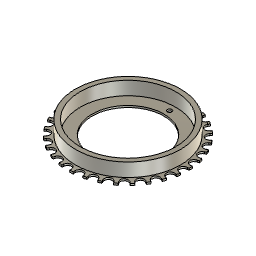
Big gear (Autodesk Fusion 360 design; units mm, degrees)
Autodesk Fusion 360 part; units mm, degrees
note: some values were not read from the file. Set by a fixed rule: which sketch regions a step uses.
sketch "Sketch1" plane through (0, 0, 0) normal (0, 1, 0) x (1, 0, 0)
sketch "Sketch2" plane through (0, 0, 0) normal (0, 0, 1) x (1, 0, 0)
  circle A0 centre (0, 0) radius 64.6805
  circle A1 centre (27.4355, 58.5735) radius 4.5
  circle A2 centre (15.4812, 62.8005) radius 4.5
  circle A3 centre (0, 0) radius 64.6805
  circle A4 centre (2.932, 64.614) radius 4.5
  circle A5 centre (0, 0) radius 64.6805
  circle A6 centre (-9.7299, 63.9445) radius 4.5
  circle A7 centre (0, 0) radius 64.6805
  circle A8 centre (-22.0179, 60.8176) radius 4.5
  circle A9 centre (0, 0) radius 64.6805
  circle A10 centre (-33.4597, 55.3535) radius 4.5
  circle A11 centre (0, 0) radius 64.6805
  circle A12 centre (-43.6158, 47.7623) radius 4.5
  circle A13 centre (0, 0) radius 64.6805
  circle A14 centre (-52.0956, 38.3355) radius 4.5
  circle A15 centre (0, 0) radius 64.6805
  circle A16 centre (-58.5735, 27.4355) radius 4.5
  circle A17 centre (0, 0) radius 64.6805
  circle A18 centre (-62.8005, 15.4812) radius 4.5
  circle A19 centre (0, 0) radius 64.6805
  circle A20 centre (-64.614, 2.932) radius 4.5
  circle A21 centre (0, 0) radius 64.6805
  circle A22 centre (-63.9445, -9.7299) radius 4.5
  circle A23 centre (-60.8176, -22.0179) radius 4.5
  circle A24 centre (0, 0) radius 64.6805
  circle A25 centre (-55.3535, -33.4597) radius 4.5
  circle A26 centre (0, 0) radius 64.6805
  circle A27 centre (-47.7623, -43.6158) radius 4.5
  circle A28 centre (0, 0) radius 64.6805
  circle A29 centre (-38.3355, -52.0956) radius 4.5
  circle A30 centre (-27.4355, -58.5735) radius 4.5
  circle A31 centre (0, 0) radius 64.6805
  circle A32 centre (-15.4812, -62.8005) radius 4.5
  circle A33 centre (0, 0) radius 64.6805
  circle A34 centre (-2.932, -64.614) radius 4.5
  circle A35 centre (0, 0) radius 64.6805
  circle A36 centre (9.7299, -63.9445) radius 4.5
  circle A37 centre (0, 0) radius 64.6805
  circle A38 centre (22.0179, -60.8176) radius 4.5
  circle A39 centre (0, 0) radius 64.6805
  circle A40 centre (33.4597, -55.3535) radius 4.5
  circle A41 centre (0, 0) radius 64.6805
  circle A42 centre (43.6158, -47.7623) radius 4.5
  circle A43 centre (0, 0) radius 64.6805
  circle A44 centre (52.0956, -38.3355) radius 4.5
  circle A45 centre (0, 0) radius 64.6805
  circle A46 centre (58.5735, -27.4355) radius 4.5
  circle A47 centre (0, 0) radius 64.6805
  circle A48 centre (62.8005, -15.4812) radius 4.5
  circle A49 centre (0, 0) radius 64.6805
  circle A50 centre (64.614, -2.932) radius 4.5
  circle A51 centre (0, 0) radius 64.6805
  circle A52 centre (63.9445, 9.7299) radius 4.5
  circle A53 centre (0, 0) radius 64.6805
  circle A54 centre (60.8176, 22.0179) radius 4.5
  circle A55 centre (0, 0) radius 64.6805
  circle A56 centre (55.3535, 33.4597) radius 4.5
  circle A57 centre (0, 0) radius 64.6805
  circle A58 centre (47.7623, 43.6158) radius 4.5
  circle A59 centre (0, 0) radius 64.6805
  circle A60 centre (38.3355, 52.0956) radius 4.5
  circle A61 centre (0, 0) radius 64.6805
  line L0 (31.4418, 56.5242) -> (34.7024, 54.583)
  line L1 (31.4418, 56.5242) -> (34.7024, 54.583)
  line L2 (31.4418, 56.5242) -> (32.4649, 58.2427)
  line L3 (32.4649, 58.2427) -> (35.6253, 56.3612)
  line L4 (35.6253, 56.3612) -> (34.5825, 54.6591)
  line L5 (19.8103, 61.5721) -> (20.4785, 63.4571)
  line L6 (20.4785, 63.4571) -> (23.9452, 62.2284)
  line L7 (23.9452, 62.2284) -> (23.2546, 60.3555)
  line L8 (7.4176, 64.2538) -> (7.7051, 66.233)
  line L9 (7.7051, 66.233) -> (11.3449, 65.7042)
  line L10 (11.3449, 65.7042) -> (11.033, 63.7326)
  line L11 (-5.2602, 64.4662) -> (-5.3643, 66.4635)
  line L12 (-5.3643, 66.4635) -> (-1.6913, 66.655)
  line L13 (-1.6913, 66.655) -> (-1.6126, 64.6604)
  line L14 (-17.7359, 62.2013) -> (-18.2277, 64.1399)
  line L15 (-18.2277, 64.1399) -> (-14.6626, 65.0443)
  line L16 (-14.6626, 65.0443) -> (-14.1963, 63.1034)
  line L17 (-29.53, 57.546) -> (-30.3905, 59.3515)
  line L18 (-30.3905, 59.3515) -> (-27.0703, 60.9339)
  line L19 (-27.0703, 60.9339) -> (-26.2343, 59.1213)
  line L20 (-40.1893, 50.6793) -> (-41.3855, 52.2821)
  line L21 (-41.3855, 52.2821) -> (-38.4378, 54.482)
  line L22 (-38.4378, 54.482) -> (-37.2642, 52.8672)
  line L23 (-49.3041, 41.865) -> (-50.79, 43.2036)
  line L24 (-50.79, 43.2036) -> (-48.3281, 45.9363)
  line L25 (-48.3281, 45.9363) -> (-46.8621, 44.5815)
  line L26 (-56.5242, 31.4418) -> (-58.2427, 32.4649)
  line L27 (-58.2427, 32.4649) -> (-56.3612, 35.6253)
  line L28 (-56.3612, 35.6253) -> (-54.6591, 34.5825)
  line L29 (-61.5721, 19.8103) -> (-63.4571, 20.4785)
  line L30 (-63.4571, 20.4785) -> (-62.2284, 23.9452)
  line L31 (-62.2284, 23.9452) -> (-60.3555, 23.2546)
  line L32 (-64.2538, 7.4176) -> (-66.233, 7.7051)
  line L33 (-66.233, 7.7051) -> (-65.7042, 11.3449)
  line L34 (-65.7042, 11.3449) -> (-63.7326, 11.033)
  line L35 (-64.4662, -5.2602) -> (-66.4635, -5.3643)
  line L36 (-66.4635, -5.3643) -> (-66.655, -1.6913)
  line L37 (-66.655, -1.6913) -> (-64.6604, -1.6126)
  line L38 (-62.2013, -17.7359) -> (-64.1399, -18.2277)
  line L39 (-64.1399, -18.2277) -> (-65.0443, -14.6626)
  line L40 (-65.0443, -14.6626) -> (-63.1034, -14.1963)
  line L41 (-57.546, -29.53) -> (-59.3515, -30.3905)
  line L42 (-59.3515, -30.3905) -> (-60.9339, -27.0703)
  line L43 (-60.9339, -27.0703) -> (-59.1213, -26.2343)
  line L44 (-50.6793, -40.1893) -> (-52.2821, -41.3855)
  line L45 (-52.2821, -41.3855) -> (-54.482, -38.4378)
  line L46 (-54.482, -38.4378) -> (-52.8672, -37.2642)
  line L47 (-41.865, -49.3041) -> (-43.2036, -50.79)
  line L48 (-43.2036, -50.79) -> (-45.9363, -48.3281)
  line L49 (-45.9363, -48.3281) -> (-44.5815, -46.8621)
  line L50 (-31.4418, -56.5242) -> (-32.4649, -58.2427)
  line L51 (-32.4649, -58.2427) -> (-35.6253, -56.3612)
  line L52 (-35.6253, -56.3612) -> (-34.5825, -54.6591)
  line L53 (-19.8103, -61.5721) -> (-20.4785, -63.4571)
  line L54 (-20.4785, -63.4571) -> (-23.9452, -62.2284)
  line L55 (-23.9452, -62.2284) -> (-23.2546, -60.3555)
  line L56 (-7.4176, -64.2538) -> (-7.7051, -66.233)
  line L57 (-7.7051, -66.233) -> (-11.3449, -65.7042)
  line L58 (-11.3449, -65.7042) -> (-11.033, -63.7326)
  line L59 (5.2602, -64.4662) -> (5.3643, -66.4635)
  line L60 (5.3643, -66.4635) -> (1.6913, -66.655)
  line L61 (1.6913, -66.655) -> (1.6126, -64.6604)
  line L62 (17.7359, -62.2013) -> (18.2277, -64.1399)
  line L63 (18.2277, -64.1399) -> (14.6626, -65.0443)
  line L64 (14.6626, -65.0443) -> (14.1963, -63.1034)
  line L65 (29.53, -57.546) -> (30.3905, -59.3515)
  line L66 (30.3905, -59.3515) -> (27.0703, -60.9339)
  line L67 (27.0703, -60.9339) -> (26.2343, -59.1213)
  line L68 (40.1893, -50.6793) -> (41.3855, -52.2821)
  line L69 (41.3855, -52.2821) -> (38.4378, -54.482)
  line L70 (38.4378, -54.482) -> (37.2642, -52.8672)
  line L71 (49.3041, -41.865) -> (50.79, -43.2036)
  line L72 (50.79, -43.2036) -> (48.3281, -45.9363)
  line L73 (48.3281, -45.9363) -> (46.8621, -44.5815)
  line L74 (56.5242, -31.4418) -> (58.2427, -32.4649)
  line L75 (58.2427, -32.4649) -> (56.3612, -35.6253)
  line L76 (56.3612, -35.6253) -> (54.6591, -34.5825)
  line L77 (61.5721, -19.8103) -> (63.4571, -20.4785)
  line L78 (63.4571, -20.4785) -> (62.2284, -23.9452)
  line L79 (62.2284, -23.9452) -> (60.3555, -23.2546)
  line L80 (64.2538, -7.4176) -> (66.233, -7.7051)
  line L81 (66.233, -7.7051) -> (65.7042, -11.3449)
  line L82 (65.7042, -11.3449) -> (63.7326, -11.033)
  line L83 (64.4662, 5.2602) -> (66.4635, 5.3643)
  line L84 (66.4635, 5.3643) -> (66.655, 1.6913)
  line L85 (66.655, 1.6913) -> (64.6604, 1.6126)
  line L86 (62.2013, 17.7359) -> (64.1399, 18.2277)
  line L87 (64.1399, 18.2277) -> (65.0443, 14.6626)
  line L88 (65.0443, 14.6626) -> (63.1034, 14.1963)
  line L89 (57.546, 29.53) -> (59.3515, 30.3905)
  line L90 (59.3515, 30.3905) -> (60.9339, 27.0703)
  line L91 (60.9339, 27.0703) -> (59.1213, 26.2343)
  line L92 (50.6793, 40.1893) -> (52.2821, 41.3855)
  line L93 (52.2821, 41.3855) -> (54.482, 38.4378)
  line L94 (54.482, 38.4378) -> (52.8672, 37.2642)
  line L95 (41.865, 49.3041) -> (43.2036, 50.79)
  line L96 (43.2036, 50.79) -> (45.9363, 48.3281)
  line L97 (45.9363, 48.3281) -> (44.5815, 46.8621)
  dimension "d1" = 129.361
  dimension "d2" = 9
  dimension "d4" = 360
  dimension "d6" = 2
  dimension "d8" = 360
  constraint coincident A0.centre A3.centre
  constraint coincident A0 A1.centre
  constraint coincident A33 L0.start
  constraint coincident A1 L0.start
  constraint coincident A31 L0.end
  constraint coincident A28 L0.end
  constraint perpendicular L1 L2
  constraint perpendicular L2 L3
  constraint coincident A59 L4.end
  constraint coincident A13 L4.end
  measures "d1" diameter of A0
  measures "d2" diameter of A1
  measures "d6" distance of L0.start L2.end
extrude "Extrude1" add sketch "Sketch2" along normal blind 2 contours A0 A1 A2 A3 A4 A5 A6 A7 A8 A9 A10 A11 A12 A13 A14 A15 A16 A17 A18 A19 A20 A21 A22 A23 A24 A25 A26 A27 A28 A29 A30 A31 A32 A33 A34 A35 A36 A37 A38 A39 A40 A41 A42 A43 A44 A45 A46 A47 A48 A49 A50 A51 A52 A53 A54 A55 A56 A57 A58 A59 A60 A61 L0 L1 | A0 A3 A5 A7 A9 A11 A13 A15 A17 A19 A21 A24 A26 A28 A31 A33 A35 A37 A39 A41 A43 A45 A47 A49 A51 A53 A55 A57 A59 A61 L83 L84 L85 | A0 A3 A5 A7 A9 A11 A13 A15 A17 A19 A21 A24 A26 A28 A31 A33 A35 A37 A39 A41 A43 A45 A47 A49 A51 A53 A55 A57 A59 A61 L80 L81 L82 | A0 A3 A5 A7 A9 A11 A13 A15 A17 A19 A21 A24 A26 A28 A31 A33 A35 A37 A39 A41 A43 A45 A47 A49 A51 A53 A55 A57 A59 A61 L86 L87 L88 | A0 A3 A5 A7 A9 A11 A13 A15 A17 A19 A21 A24 A26 A28 A31 A33 A35 A37 A39 A41 A43 A45 A47 A49 A51 A53 A55 A57 A59 A61 L77 L78 L79 | A0 A3 A5 A7 A9 A11 A13 A15 A17 A19 A21 A24 A26 A28 A31 A33 A35 A37 A39 A41 A43 A45 A47 A49 A51 A53 A55 A57 A59 A61 L89 L90 L91 | A0 A3 A5 A7 A9 A11 A13 A15 A17 A19 A21 A24 A26 A28 A31 A33 A35 A37 A39 A41 A43 A45 A47 A49 A51 A53 A55 A57 A59 A61 L74 L75 L76 | A0 A3 A5 A7 A9 A11 A13 A15 A17 A19 A21 A24 A26 A28 A31 A33 A35 A37 A39 A41 A43 A45 A47 A49 A51 A53 A55 A57 A59 A61 L92 L93 L94 | A0 A3 A5 A7 A9 A11 A13 A15 A17 A19 A21 A24 A26 A28 A31 A33 A35 A37 A39 A41 A43 A45 A47 A49 A51 A53 A55 A57 A59 A61 L71 L72 L73 | A0 A3 A5 A7 A9 A11 A13 A15 A17 A19 A21 A24 A26 A28 A31 A33 A35 A37 A39 A41 A43 A45 A47 A49 A51 A53 A55 A57 A59 A61 L95 L96 L97 | A0 A3 A5 A7 A9 A11 A13 A15 A17 A19 A21 A24 A26 A28 A31 A33 A35 A37 A39 A41 A43 A45 A47 A49 A51 A53 A55 A57 A59 A61 L68 L69 L70 | A0 A3 A5 A7 A9 A11 A13 A15 A17 A19 A21 A24 A26 A28 A31 A33 A35 A37 A39 A41 A43 A45 A47 A49 A51 A53 A55 A57 A59 A61 L2 L3 L4 | A0 A3 A5 A7 A9 A11 A13 A15 A17 A19 A21 A24 A26 A28 A31 A33 A35 A37 A39 A41 A43 A45 A47 A49 A51 A53 A55 A57 A59 A61 L5 L6 L7 | A0 A3 A5 A7 A9 A11 A13 A15 A17 A19 A21 A24 A26 A28 A31 A33 A35 A37 A39 A41 A43 A45 A47 A49 A51 A53 A55 A57 A59 A61 L65 L66 L67 | A0 A3 A5 A7 A9 A11 A13 A15 A17 A19 A21 A24 A26 A28 A31 A33 A35 A37 A39 A41 A43 A45 A47 A49 A51 A53 A55 A57 A59 A61 L8 L9 L10 | A0 A3 A5 A7 A9 A11 A13 A15 A17 A19 A21 A24 A26 A28 A31 A33 A35 A37 A39 A41 A43 A45 A47 A49 A51 A53 A55 A57 A59 A61 L62 L63 L64 | A0 A3 A5 A7 A9 A11 A13 A15 A17 A19 A21 A24 A26 A28 A31 A33 A35 A37 A39 A41 A43 A45 A47 A49 A51 A53 A55 A57 A59 A61 L11 L12 L13 | A0 A3 A5 A7 A9 A11 A13 A15 A17 A19 A21 A24 A26 A28 A31 A33 A35 A37 A39 A41 A43 A45 A47 A49 A51 A53 A55 A57 A59 A61 L59 L60 L61 | A0 A3 A5 A7 A9 A11 A13 A15 A17 A19 A21 A24 A26 A28 A31 A33 A35 A37 A39 A41 A43 A45 A47 A49 A51 A53 A55 A57 A59 A61 L14 L15 L16 | A0 A3 A5 A7 A9 A11 A13 A15 A17 A19 A21 A24 A26 A28 A31 A33 A35 A37 A39 A41 A43 A45 A47 A49 A51 A53 A55 A57 A59 A61 L56 L57 L58 | A0 A3 A5 A7 A9 A11 A13 A15 A17 A19 A21 A24 A26 A28 A31 A33 A35 A37 A39 A41 A43 A45 A47 A49 A51 A53 A55 A57 A59 A61 L17 L18 L19 | A0 A3 A5 A7 A9 A11 A13 A15 A17 A19 A21 A24 A26 A28 A31 A33 A35 A37 A39 A41 A43 A45 A47 A49 A51 A53 A55 A57 A59 A61 L53 L54 L55 | A0 A3 A5 A7 A9 A11 A13 A15 A17 A19 A21 A24 A26 A28 A31 A33 A35 A37 A39 A41 A43 A45 A47 A49 A51 A53 A55 A57 A59 A61 L20 L21 L22 | A0 A3 A5 A7 A9 A11 A13 A15 A17 A19 A21 A24 A26 A28 A31 A33 A35 A37 A39 A41 A43 A45 A47 A49 A51 A53 A55 A57 A59 A61 L50 L51 L52 | A0 A3 A5 A7 A9 A11 A13 A15 A17 A19 A21 A24 A26 A28 A31 A33 A35 A37 A39 A41 A43 A45 A47 A49 A51 A53 A55 A57 A59 A61 L23 L24 L25 | A0 A3 A5 A7 A9 A11 A13 A15 A17 A19 A21 A24 A26 A28 A31 A33 A35 A37 A39 A41 A43 A45 A47 A49 A51 A53 A55 A57 A59 A61 L47 L48 L49 | A0 A3 A5 A7 A9 A11 A13 A15 A17 A19 A21 A24 A26 A28 A31 A33 A35 A37 A39 A41 A43 A45 A47 A49 A51 A53 A55 A57 A59 A61 L26 L27 L28 | A0 A3 A5 A7 A9 A11 A13 A15 A17 A19 A21 A24 A26 A28 A31 A33 A35 A37 A39 A41 A43 A45 A47 A49 A51 A53 A55 A57 A59 A61 L44 L45 L46 | A0 A3 A5 A7 A9 A11 A13 A15 A17 A19 A21 A24 A26 A28 A31 A33 A35 A37 A39 A41 A43 A45 A47 A49 A51 A53 A55 A57 A59 A61 L29 L30 L31 | A0 A3 A5 A7 A9 A11 A13 A15 A17 A19 A21 A24 A26 A28 A31 A33 A35 A37 A39 A41 A43 A45 A47 A49 A51 A53 A55 A57 A59 A61 L41 L42 L43 | A0 A3 A5 A7 A9 A11 A13 A15 A17 A19 A21 A24 A26 A28 A31 A33 A35 A37 A39 A41 A43 A45 A47 A49 A51 A53 A55 A57 A59 A61 L32 L33 L34 | A0 A3 A5 A7 A9 A11 A13 A15 A17 A19 A21 A24 A26 A28 A31 A33 A35 A37 A39 A41 A43 A45 A47 A49 A51 A53 A55 A57 A59 A61 L38 L39 L40 | A0 A3 A5 A7 A9 A11 A13 A15 A17 A19 A21 A24 A26 A28 A31 A33 A35 A37 A39 A41 A43 A45 A47 A49 A51 A53 A55 A57 A59 A61 L35 L36 L37 makes body 1 at (-8.6099, -18.1233, 0)
sketch "Sketch9" plane through (0, 0, 2) normal (0, 0, 1) x (-1, 0, 0)
  arc A0 (-23.2965, -60.3394) -> (-23.2546, -60.3555) centre (0, 0) ccw
  line L0 (-23.2546, -60.3555) -> (-23.9452, -62.2284)
  line L1 (-23.9452, -62.2284) -> (-20.4785, -63.4571)
  line L2 (-20.4785, -63.4571) -> (-19.8103, -61.5721)
  arc A1 (-11.0772, -63.7249) -> (-19.8103, -61.5721) centre (-15.4812, -62.8005) ccw
  arc A2 (-11.0772, -63.7249) -> (-11.033, -63.7326) centre (0, 0) ccw
  line L3 (-11.033, -63.7326) -> (-11.3449, -65.7042)
  line L4 (-11.3449, -65.7042) -> (-7.7051, -66.233)
  line L5 (-7.7051, -66.233) -> (-7.4176, -64.2538)
  arc A3 (1.5677, -64.6615) -> (-7.4176, -64.2538) centre (-2.932, -64.614) ccw
  arc A4 (1.5677, -64.6615) -> (1.6126, -64.6604) centre (0, 0) ccw
  line L6 (1.6126, -64.6604) -> (1.6913, -66.655)
  line L7 (1.6913, -66.655) -> (5.3643, -66.4635)
  line L8 (5.3643, -66.4635) -> (5.2602, -64.4662)
  arc A5 (14.1524, -63.1132) -> (5.2602, -64.4662) centre (9.7299, -63.9445) ccw
  arc A6 (14.1524, -63.1132) -> (14.1963, -63.1034) centre (0, 0) ccw
  line L9 (14.1963, -63.1034) -> (14.6626, -65.0443)
  line L10 (14.6626, -65.0443) -> (18.2277, -64.1399)
  line L11 (18.2277, -64.1399) -> (17.7359, -62.2013)
  arc A7 (26.1933, -59.1395) -> (17.7359, -62.2013) centre (22.0179, -60.8176) ccw
  arc A8 (26.1933, -59.1395) -> (26.2343, -59.1213) centre (0, 0) ccw
  line L12 (26.2343, -59.1213) -> (27.0703, -60.9339)
  line L13 (27.0703, -60.9339) -> (30.3905, -59.3515)
  line L14 (30.3905, -59.3515) -> (29.53, -57.546)
  arc A9 (37.2275, -52.8931) -> (29.53, -57.546) centre (33.4597, -55.3535) ccw
  arc A10 (37.2275, -52.8931) -> (37.2642, -52.8672) centre (0, 0) ccw
  line L15 (37.2642, -52.8672) -> (38.4378, -54.482)
  line L16 (38.4378, -54.482) -> (41.3855, -52.2821)
  line L17 (41.3855, -52.2821) -> (40.1893, -50.6793)
  arc A11 (46.8311, -44.614) -> (40.1893, -50.6793) centre (43.6158, -47.7623) ccw
  arc A12 (46.8311, -44.614) -> (46.8621, -44.5815) centre (0, 0) ccw
  line L18 (46.8621, -44.5815) -> (48.3281, -45.9363)
  line L19 (48.3281, -45.9363) -> (50.79, -43.2036)
  line L20 (50.79, -43.2036) -> (49.3041, -41.865)
  arc A13 (54.6351, -34.6205) -> (49.3041, -41.865) centre (52.0956, -38.3355) ccw
  arc A14 (54.6351, -34.6205) -> (54.6591, -34.5825) centre (0, 0) ccw
  line L21 (54.6591, -34.5825) -> (56.3612, -35.6253)
  line L22 (56.3612, -35.6253) -> (58.2427, -32.4649)
  line L23 (58.2427, -32.4649) -> (56.5242, -31.4418)
  arc A15 (60.3394, -23.2965) -> (56.5242, -31.4418) centre (58.5735, -27.4355) ccw
  arc A16 (60.3394, -23.2965) -> (60.3555, -23.2546) centre (0, 0) ccw
  line L24 (60.3555, -23.2546) -> (62.2284, -23.9452)
  line L25 (62.2284, -23.9452) -> (63.4571, -20.4785)
  line L26 (63.4571, -20.4785) -> (61.5721, -19.8103)
  arc A17 (63.7249, -11.0772) -> (61.5721, -19.8103) centre (62.8005, -15.4812) ccw
  arc A18 (63.7249, -11.0772) -> (63.7326, -11.033) centre (0, 0) ccw
  line L27 (63.7326, -11.033) -> (65.7042, -11.3449)
  line L28 (65.7042, -11.3449) -> (66.233, -7.7051)
  line L29 (66.233, -7.7051) -> (64.2538, -7.4176)
  arc A19 (64.6615, 1.5677) -> (64.2538, -7.4176) centre (64.614, -2.932) ccw
  arc A20 (64.6615, 1.5677) -> (64.6604, 1.6126) centre (0, 0) ccw
  line L30 (64.6604, 1.6126) -> (66.655, 1.6913)
  line L31 (66.655, 1.6913) -> (66.4635, 5.3643)
  line L32 (66.4635, 5.3643) -> (64.4662, 5.2602)
  arc A21 (63.1132, 14.1524) -> (64.4662, 5.2602) centre (63.9445, 9.7299) ccw
  arc A22 (63.1132, 14.1524) -> (63.1034, 14.1963) centre (0, 0) ccw
  line L33 (63.1034, 14.1963) -> (65.0443, 14.6626)
  line L34 (65.0443, 14.6626) -> (64.1399, 18.2277)
  line L35 (64.1399, 18.2277) -> (62.2013, 17.7359)
  arc A23 (59.1395, 26.1933) -> (62.2013, 17.7359) centre (60.8176, 22.0179) ccw
  arc A24 (59.1395, 26.1933) -> (59.1213, 26.2343) centre (0, 0) ccw
  line L36 (59.1213, 26.2343) -> (60.9339, 27.0703)
  line L37 (60.9339, 27.0703) -> (59.3515, 30.3905)
  line L38 (59.3515, 30.3905) -> (57.546, 29.53)
  arc A25 (52.8931, 37.2275) -> (57.546, 29.53) centre (55.3535, 33.4597) ccw
  arc A26 (52.8931, 37.2275) -> (52.8672, 37.2642) centre (0, 0) ccw
  line L39 (52.8672, 37.2642) -> (54.482, 38.4378)
  line L40 (54.482, 38.4378) -> (52.2821, 41.3855)
  line L41 (52.2821, 41.3855) -> (50.6793, 40.1893)
  arc A27 (44.614, 46.8311) -> (50.6793, 40.1893) centre (47.7623, 43.6158) ccw
  arc A28 (44.614, 46.8311) -> (44.5815, 46.8621) centre (0, 0) ccw
  line L42 (44.5815, 46.8621) -> (45.9363, 48.3281)
  line L43 (45.9363, 48.3281) -> (43.2036, 50.79)
  line L44 (43.2036, 50.79) -> (41.865, 49.3041)
  arc A29 (34.6205, 54.6351) -> (41.865, 49.3041) centre (38.3355, 52.0956) ccw
  arc A30 (34.6205, 54.6351) -> (34.5825, 54.6591) centre (0, 0) ccw
  line L45 (34.5825, 54.6591) -> (35.6253, 56.3612)
  line L46 (35.6253, 56.3612) -> (32.4649, 58.2427)
  line L47 (32.4649, 58.2427) -> (31.4418, 56.5242)
  arc A31 (23.2965, 60.3394) -> (31.4418, 56.5242) centre (27.4355, 58.5735) ccw
  arc A32 (23.2965, 60.3394) -> (23.2546, 60.3555) centre (0, 0) ccw
  line L48 (23.2546, 60.3555) -> (23.9452, 62.2284)
  line L49 (23.9452, 62.2284) -> (20.4785, 63.4571)
  line L50 (20.4785, 63.4571) -> (19.8103, 61.5721)
  arc A33 (11.0772, 63.7249) -> (19.8103, 61.5721) centre (15.4812, 62.8005) ccw
  arc A34 (11.0772, 63.7249) -> (11.033, 63.7326) centre (0, 0) ccw
  line L51 (11.033, 63.7326) -> (11.3449, 65.7042)
  line L52 (11.3449, 65.7042) -> (7.7051, 66.233)
  line L53 (7.7051, 66.233) -> (7.4176, 64.2538)
  arc A35 (-1.5677, 64.6615) -> (7.4176, 64.2538) centre (2.932, 64.614) ccw
  arc A36 (-1.5677, 64.6615) -> (-1.6126, 64.6604) centre (0, 0) ccw
  line L54 (-1.6126, 64.6604) -> (-1.6913, 66.655)
  line L55 (-1.6913, 66.655) -> (-5.3643, 66.4635)
  line L56 (-5.3643, 66.4635) -> (-5.2602, 64.4662)
  arc A37 (-14.1524, 63.1132) -> (-5.2602, 64.4662) centre (-9.7299, 63.9445) ccw
  arc A38 (-14.1524, 63.1132) -> (-14.1963, 63.1034) centre (0, 0) ccw
  line L57 (-14.1963, 63.1034) -> (-14.6626, 65.0443)
  line L58 (-14.6626, 65.0443) -> (-18.2277, 64.1399)
  line L59 (-18.2277, 64.1399) -> (-17.7359, 62.2013)
  arc A39 (-26.1933, 59.1395) -> (-17.7359, 62.2013) centre (-22.0179, 60.8176) ccw
  arc A40 (-26.1933, 59.1395) -> (-26.2343, 59.1213) centre (0, 0) ccw
  line L60 (-26.2343, 59.1213) -> (-27.0703, 60.9339)
  line L61 (-27.0703, 60.9339) -> (-30.3905, 59.3515)
  line L62 (-30.3905, 59.3515) -> (-29.53, 57.546)
  arc A41 (-37.2275, 52.8931) -> (-29.53, 57.546) centre (-33.4597, 55.3535) ccw
  arc A42 (-37.2275, 52.8931) -> (-37.2642, 52.8672) centre (0, 0) ccw
  line L63 (-37.2642, 52.8672) -> (-38.4378, 54.482)
  line L64 (-38.4378, 54.482) -> (-41.3855, 52.2821)
  line L65 (-41.3855, 52.2821) -> (-40.1893, 50.6793)
  arc A43 (-46.8311, 44.614) -> (-40.1893, 50.6793) centre (-43.6158, 47.7623) ccw
  arc A44 (-46.8311, 44.614) -> (-46.8621, 44.5815) centre (0, 0) ccw
  line L66 (-46.8621, 44.5815) -> (-48.3281, 45.9363)
  line L67 (-48.3281, 45.9363) -> (-50.79, 43.2036)
  line L68 (-50.79, 43.2036) -> (-49.3041, 41.865)
  arc A45 (-54.6351, 34.6205) -> (-49.3041, 41.865) centre (-52.0956, 38.3355) ccw
  arc A46 (-54.6351, 34.6205) -> (-54.6591, 34.5825) centre (0, 0) ccw
  line L69 (-54.6591, 34.5825) -> (-56.3612, 35.6253)
  line L70 (-56.3612, 35.6253) -> (-58.2427, 32.4649)
  line L71 (-58.2427, 32.4649) -> (-56.5242, 31.4418)
  arc A47 (-60.3394, 23.2965) -> (-56.5242, 31.4418) centre (-58.5735, 27.4355) ccw
  arc A48 (-60.3394, 23.2965) -> (-60.3555, 23.2546) centre (0, 0) ccw
  line L72 (-60.3555, 23.2546) -> (-62.2284, 23.9452)
  line L73 (-62.2284, 23.9452) -> (-63.4571, 20.4785)
  line L74 (-63.4571, 20.4785) -> (-61.5721, 19.8103)
  arc A49 (-63.7249, 11.0772) -> (-61.5721, 19.8103) centre (-62.8005, 15.4812) ccw
  arc A50 (-63.7249, 11.0772) -> (-63.7326, 11.033) centre (0, 0) ccw
  line L75 (-63.7326, 11.033) -> (-65.7042, 11.3449)
  line L76 (-65.7042, 11.3449) -> (-66.233, 7.7051)
  line L77 (-66.233, 7.7051) -> (-64.2538, 7.4176)
  arc A51 (-64.6615, -1.5677) -> (-64.2538, 7.4176) centre (-64.614, 2.932) ccw
  arc A52 (-64.6615, -1.5677) -> (-64.6604, -1.6126) centre (0, 0) ccw
  line L78 (-64.6604, -1.6126) -> (-66.655, -1.6913)
  line L79 (-66.655, -1.6913) -> (-66.4635, -5.3643)
  line L80 (-66.4635, -5.3643) -> (-64.4662, -5.2602)
  arc A53 (-63.1132, -14.1524) -> (-64.4662, -5.2602) centre (-63.9445, -9.7299) ccw
  arc A54 (-63.1132, -14.1524) -> (-63.1034, -14.1963) centre (0, 0) ccw
  line L81 (-63.1034, -14.1963) -> (-65.0443, -14.6626)
  line L82 (-65.0443, -14.6626) -> (-64.1399, -18.2277)
  line L83 (-64.1399, -18.2277) -> (-62.2013, -17.7359)
  arc A55 (-59.1395, -26.1933) -> (-62.2013, -17.7359) centre (-60.8176, -22.0179) ccw
  arc A56 (-59.1395, -26.1933) -> (-59.1213, -26.2343) centre (0, 0) ccw
  line L84 (-59.1213, -26.2343) -> (-60.9339, -27.0703)
  line L85 (-60.9339, -27.0703) -> (-59.3515, -30.3905)
  line L86 (-59.3515, -30.3905) -> (-57.546, -29.53)
  arc A57 (-52.8931, -37.2275) -> (-57.546, -29.53) centre (-55.3535, -33.4597) ccw
  arc A58 (-52.8931, -37.2275) -> (-52.8672, -37.2642) centre (0, 0) ccw
  line L87 (-52.8672, -37.2642) -> (-54.482, -38.4378)
  line L88 (-54.482, -38.4378) -> (-52.2821, -41.3855)
  line L89 (-52.2821, -41.3855) -> (-50.6793, -40.1893)
  arc A59 (-44.614, -46.8311) -> (-50.6793, -40.1893) centre (-47.7623, -43.6158) ccw
  arc A60 (-44.614, -46.8311) -> (-44.5815, -46.8621) centre (0, 0) ccw
  line L90 (-44.5815, -46.8621) -> (-45.9363, -48.3281)
  line L91 (-45.9363, -48.3281) -> (-43.2036, -50.79)
  line L92 (-43.2036, -50.79) -> (-41.865, -49.3041)
  arc A61 (-34.6189, -54.6328) -> (-41.865, -49.3041) centre (-38.3355, -52.0956) ccw
  line L93 (-34.6189, -54.6328) -> (-31.4418, -56.5242)
  arc A62 (-23.2965, -60.3394) -> (-31.4418, -56.5242) centre (-27.4355, -58.5735) ccw
  circle A63 centre (0, 0) radius 40
  circle A64 centre (0, -46.5) radius 2.5
  circle A65 centre (0.1887, 46.5) radius 2.5
  dimension "d27" = 80
  dimension "d28" = 5
  dimension "d29" = 5
  dimension "d30" = 46.5
  dimension "d31" = 46.5
  constraint coincident A0.centre A2.centre
  measures "d27" diameter of A63
  measures "d28" diameter of A64
  measures "d29" diameter of A65
  measures "d30" distance of A0.centre A64.centre
  measures "d31" vertical distance of A0.centre A65.centre
extrude "Extrude7" cut sketch "Sketch9" against normal blind 3 contours A63 | A64 | A65 bodies 1
sketch "Sketch10" plane through (0, 0, 2) normal (0, 0, 1) x (-1, 0, 0)
  circle A0 centre (0, -46.5) radius 2.5
  circle A1 centre (0, 0) radius 40
  circle A2 centre (0.1887, 46.5) radius 2.5
  arc A3 (-23.2965, -60.3394) -> (-23.2546, -60.3555) centre (0, 0) ccw
  line L0 (-23.2546, -60.3555) -> (-23.9452, -62.2284)
  line L1 (-23.9452, -62.2284) -> (-20.4785, -63.4571)
  line L2 (-20.4785, -63.4571) -> (-19.8103, -61.5721)
  arc A4 (-11.0772, -63.7249) -> (-19.8103, -61.5721) centre (-15.4812, -62.8005) ccw
  arc A5 (-11.0772, -63.7249) -> (-11.033, -63.7326) centre (0, 0) ccw
  line L3 (-11.033, -63.7326) -> (-11.3449, -65.7042)
  line L4 (-11.3449, -65.7042) -> (-7.7051, -66.233)
  line L5 (-7.7051, -66.233) -> (-7.4176, -64.2538)
  arc A6 (1.5677, -64.6615) -> (-7.4176, -64.2538) centre (-2.932, -64.614) ccw
  arc A7 (1.5677, -64.6615) -> (1.6126, -64.6604) centre (0, 0) ccw
  line L6 (1.6126, -64.6604) -> (1.6913, -66.655)
  line L7 (1.6913, -66.655) -> (5.3643, -66.4635)
  line L8 (5.3643, -66.4635) -> (5.2602, -64.4662)
  arc A8 (14.1524, -63.1132) -> (5.2602, -64.4662) centre (9.7299, -63.9445) ccw
  arc A9 (14.1524, -63.1132) -> (14.1963, -63.1034) centre (0, 0) ccw
  line L9 (14.1963, -63.1034) -> (14.6626, -65.0443)
  line L10 (14.6626, -65.0443) -> (18.2277, -64.1399)
  line L11 (18.2277, -64.1399) -> (17.7359, -62.2013)
  arc A10 (26.1933, -59.1395) -> (17.7359, -62.2013) centre (22.0179, -60.8176) ccw
  arc A11 (26.1933, -59.1395) -> (26.2343, -59.1213) centre (0, 0) ccw
  line L12 (26.2343, -59.1213) -> (27.0703, -60.9339)
  line L13 (27.0703, -60.9339) -> (30.3905, -59.3515)
  line L14 (30.3905, -59.3515) -> (29.53, -57.546)
  arc A12 (37.2275, -52.8931) -> (29.53, -57.546) centre (33.4597, -55.3535) ccw
  arc A13 (37.2275, -52.8931) -> (37.2642, -52.8672) centre (0, 0) ccw
  line L15 (37.2642, -52.8672) -> (38.4378, -54.482)
  line L16 (38.4378, -54.482) -> (41.3855, -52.2821)
  line L17 (41.3855, -52.2821) -> (40.1893, -50.6793)
  arc A14 (46.8311, -44.614) -> (40.1893, -50.6793) centre (43.6158, -47.7623) ccw
  arc A15 (46.8311, -44.614) -> (46.8621, -44.5815) centre (0, 0) ccw
  line L18 (46.8621, -44.5815) -> (48.3281, -45.9363)
  line L19 (48.3281, -45.9363) -> (50.79, -43.2036)
  line L20 (50.79, -43.2036) -> (49.3041, -41.865)
  arc A16 (54.6351, -34.6205) -> (49.3041, -41.865) centre (52.0956, -38.3355) ccw
  arc A17 (54.6351, -34.6205) -> (54.6591, -34.5825) centre (0, 0) ccw
  line L21 (54.6591, -34.5825) -> (56.3612, -35.6253)
  line L22 (56.3612, -35.6253) -> (58.2427, -32.4649)
  line L23 (58.2427, -32.4649) -> (56.5242, -31.4418)
  arc A18 (60.3394, -23.2965) -> (56.5242, -31.4418) centre (58.5735, -27.4355) ccw
  arc A19 (60.3394, -23.2965) -> (60.3555, -23.2546) centre (0, 0) ccw
  line L24 (60.3555, -23.2546) -> (62.2284, -23.9452)
  line L25 (62.2284, -23.9452) -> (63.4571, -20.4785)
  line L26 (63.4571, -20.4785) -> (61.5721, -19.8103)
  arc A20 (63.7249, -11.0772) -> (61.5721, -19.8103) centre (62.8005, -15.4812) ccw
  arc A21 (63.7249, -11.0772) -> (63.7326, -11.033) centre (0, 0) ccw
  line L27 (63.7326, -11.033) -> (65.7042, -11.3449)
  line L28 (65.7042, -11.3449) -> (66.233, -7.7051)
  line L29 (66.233, -7.7051) -> (64.2538, -7.4176)
  arc A22 (64.6615, 1.5677) -> (64.2538, -7.4176) centre (64.614, -2.932) ccw
  arc A23 (64.6615, 1.5677) -> (64.6604, 1.6126) centre (0, 0) ccw
  line L30 (64.6604, 1.6126) -> (66.655, 1.6913)
  line L31 (66.655, 1.6913) -> (66.4635, 5.3643)
  line L32 (66.4635, 5.3643) -> (64.4662, 5.2602)
  arc A24 (63.1132, 14.1524) -> (64.4662, 5.2602) centre (63.9445, 9.7299) ccw
  arc A25 (63.1132, 14.1524) -> (63.1034, 14.1963) centre (0, 0) ccw
  line L33 (63.1034, 14.1963) -> (65.0443, 14.6626)
  line L34 (65.0443, 14.6626) -> (64.1399, 18.2277)
  line L35 (64.1399, 18.2277) -> (62.2013, 17.7359)
  arc A26 (59.1395, 26.1933) -> (62.2013, 17.7359) centre (60.8176, 22.0179) ccw
  arc A27 (59.1395, 26.1933) -> (59.1213, 26.2343) centre (0, 0) ccw
  line L36 (59.1213, 26.2343) -> (60.9339, 27.0703)
  line L37 (60.9339, 27.0703) -> (59.3515, 30.3905)
  line L38 (59.3515, 30.3905) -> (57.546, 29.53)
  arc A28 (52.8931, 37.2275) -> (57.546, 29.53) centre (55.3535, 33.4597) ccw
  arc A29 (52.8931, 37.2275) -> (52.8672, 37.2642) centre (0, 0) ccw
  line L39 (52.8672, 37.2642) -> (54.482, 38.4378)
  line L40 (54.482, 38.4378) -> (52.2821, 41.3855)
  line L41 (52.2821, 41.3855) -> (50.6793, 40.1893)
  arc A30 (44.614, 46.8311) -> (50.6793, 40.1893) centre (47.7623, 43.6158) ccw
  arc A31 (44.614, 46.8311) -> (44.5815, 46.8621) centre (0, 0) ccw
  line L42 (44.5815, 46.8621) -> (45.9363, 48.3281)
  line L43 (45.9363, 48.3281) -> (43.2036, 50.79)
  line L44 (43.2036, 50.79) -> (41.865, 49.3041)
  arc A32 (34.6205, 54.6351) -> (41.865, 49.3041) centre (38.3355, 52.0956) ccw
  arc A33 (34.6205, 54.6351) -> (34.5825, 54.6591) centre (0, 0) ccw
  line L45 (34.5825, 54.6591) -> (35.6253, 56.3612)
  line L46 (35.6253, 56.3612) -> (32.4649, 58.2427)
  line L47 (32.4649, 58.2427) -> (31.4418, 56.5242)
  arc A34 (23.2965, 60.3394) -> (31.4418, 56.5242) centre (27.4355, 58.5735) ccw
  arc A35 (23.2965, 60.3394) -> (23.2546, 60.3555) centre (0, 0) ccw
  line L48 (23.2546, 60.3555) -> (23.9452, 62.2284)
  line L49 (23.9452, 62.2284) -> (20.4785, 63.4571)
  line L50 (20.4785, 63.4571) -> (19.8103, 61.5721)
  arc A36 (11.0772, 63.7249) -> (19.8103, 61.5721) centre (15.4812, 62.8005) ccw
  arc A37 (11.0772, 63.7249) -> (11.033, 63.7326) centre (0, 0) ccw
  line L51 (11.033, 63.7326) -> (11.3449, 65.7042)
  line L52 (11.3449, 65.7042) -> (7.7051, 66.233)
  line L53 (7.7051, 66.233) -> (7.4176, 64.2538)
  arc A38 (-1.5677, 64.6615) -> (7.4176, 64.2538) centre (2.932, 64.614) ccw
  arc A39 (-1.5677, 64.6615) -> (-1.6126, 64.6604) centre (0, 0) ccw
  line L54 (-1.6126, 64.6604) -> (-1.6913, 66.655)
  line L55 (-1.6913, 66.655) -> (-5.3643, 66.4635)
  line L56 (-5.3643, 66.4635) -> (-5.2602, 64.4662)
  arc A40 (-14.1524, 63.1132) -> (-5.2602, 64.4662) centre (-9.7299, 63.9445) ccw
  arc A41 (-14.1524, 63.1132) -> (-14.1963, 63.1034) centre (0, 0) ccw
  line L57 (-14.1963, 63.1034) -> (-14.6626, 65.0443)
  line L58 (-14.6626, 65.0443) -> (-18.2277, 64.1399)
  line L59 (-18.2277, 64.1399) -> (-17.7359, 62.2013)
  arc A42 (-26.1933, 59.1395) -> (-17.7359, 62.2013) centre (-22.0179, 60.8176) ccw
  arc A43 (-26.1933, 59.1395) -> (-26.2343, 59.1213) centre (0, 0) ccw
  line L60 (-26.2343, 59.1213) -> (-27.0703, 60.9339)
  line L61 (-27.0703, 60.9339) -> (-30.3905, 59.3515)
  line L62 (-30.3905, 59.3515) -> (-29.53, 57.546)
  arc A44 (-37.2275, 52.8931) -> (-29.53, 57.546) centre (-33.4597, 55.3535) ccw
  arc A45 (-37.2275, 52.8931) -> (-37.2642, 52.8672) centre (0, 0) ccw
  line L63 (-37.2642, 52.8672) -> (-38.4378, 54.482)
  line L64 (-38.4378, 54.482) -> (-41.3855, 52.2821)
  line L65 (-41.3855, 52.2821) -> (-40.1893, 50.6793)
  arc A46 (-46.8311, 44.614) -> (-40.1893, 50.6793) centre (-43.6158, 47.7623) ccw
  arc A47 (-46.8311, 44.614) -> (-46.8621, 44.5815) centre (0, 0) ccw
  line L66 (-46.8621, 44.5815) -> (-48.3281, 45.9363)
  line L67 (-48.3281, 45.9363) -> (-50.79, 43.2036)
  line L68 (-50.79, 43.2036) -> (-49.3041, 41.865)
  arc A48 (-54.6351, 34.6205) -> (-49.3041, 41.865) centre (-52.0956, 38.3355) ccw
  arc A49 (-54.6351, 34.6205) -> (-54.6591, 34.5825) centre (0, 0) ccw
  line L69 (-54.6591, 34.5825) -> (-56.3612, 35.6253)
  line L70 (-56.3612, 35.6253) -> (-58.2427, 32.4649)
  line L71 (-58.2427, 32.4649) -> (-56.5242, 31.4418)
  arc A50 (-60.3394, 23.2965) -> (-56.5242, 31.4418) centre (-58.5735, 27.4355) ccw
  arc A51 (-60.3394, 23.2965) -> (-60.3555, 23.2546) centre (0, 0) ccw
  line L72 (-60.3555, 23.2546) -> (-62.2284, 23.9452)
  line L73 (-62.2284, 23.9452) -> (-63.4571, 20.4785)
  line L74 (-63.4571, 20.4785) -> (-61.5721, 19.8103)
  arc A52 (-63.7249, 11.0772) -> (-61.5721, 19.8103) centre (-62.8005, 15.4812) ccw
  arc A53 (-63.7249, 11.0772) -> (-63.7326, 11.033) centre (0, 0) ccw
  line L75 (-63.7326, 11.033) -> (-65.7042, 11.3449)
  line L76 (-65.7042, 11.3449) -> (-66.233, 7.7051)
  line L77 (-66.233, 7.7051) -> (-64.2538, 7.4176)
  arc A54 (-64.6615, -1.5677) -> (-64.2538, 7.4176) centre (-64.614, 2.932) ccw
  arc A55 (-64.6615, -1.5677) -> (-64.6604, -1.6126) centre (0, 0) ccw
  line L78 (-64.6604, -1.6126) -> (-66.655, -1.6913)
  line L79 (-66.655, -1.6913) -> (-66.4635, -5.3643)
  line L80 (-66.4635, -5.3643) -> (-64.4662, -5.2602)
  arc A56 (-63.1132, -14.1524) -> (-64.4662, -5.2602) centre (-63.9445, -9.7299) ccw
  arc A57 (-63.1132, -14.1524) -> (-63.1034, -14.1963) centre (0, 0) ccw
  line L81 (-63.1034, -14.1963) -> (-65.0443, -14.6626)
  line L82 (-65.0443, -14.6626) -> (-64.1399, -18.2277)
  line L83 (-64.1399, -18.2277) -> (-62.2013, -17.7359)
  arc A58 (-59.1395, -26.1933) -> (-62.2013, -17.7359) centre (-60.8176, -22.0179) ccw
  arc A59 (-59.1395, -26.1933) -> (-59.1213, -26.2343) centre (0, 0) ccw
  line L84 (-59.1213, -26.2343) -> (-60.9339, -27.0703)
  line L85 (-60.9339, -27.0703) -> (-59.3515, -30.3905)
  line L86 (-59.3515, -30.3905) -> (-57.546, -29.53)
  arc A60 (-52.8931, -37.2275) -> (-57.546, -29.53) centre (-55.3535, -33.4597) ccw
  arc A61 (-52.8931, -37.2275) -> (-52.8672, -37.2642) centre (0, 0) ccw
  line L87 (-52.8672, -37.2642) -> (-54.482, -38.4378)
  line L88 (-54.482, -38.4378) -> (-52.2821, -41.3855)
  line L89 (-52.2821, -41.3855) -> (-50.6793, -40.1893)
  arc A62 (-44.614, -46.8311) -> (-50.6793, -40.1893) centre (-47.7623, -43.6158) ccw
  arc A63 (-44.614, -46.8311) -> (-44.5815, -46.8621) centre (0, 0) ccw
  line L90 (-44.5815, -46.8621) -> (-45.9363, -48.3281)
  line L91 (-45.9363, -48.3281) -> (-43.2036, -50.79)
  line L92 (-43.2036, -50.79) -> (-41.865, -49.3041)
  arc A64 (-34.6189, -54.6328) -> (-41.865, -49.3041) centre (-38.3355, -52.0956) ccw
  line L93 (-34.6189, -54.6328) -> (-31.4418, -56.5242)
  arc A65 (-23.2965, -60.3394) -> (-31.4418, -56.5242) centre (-27.4355, -58.5735) ccw
  circle A66 centre (0, 0) radius 53.25
  circle A67 centre (0, 0) radius 58.5
  dimension "d34" = 106.5
  dimension "d35" = 117
  constraint coincident A1.centre A3.centre
  constraint concentric A1 A67
  measures "d34" diameter of A66
  measures "d35" diameter of A67
extrude "Extrude8" add sketch "Sketch10" along normal blind 15 separate body contours A67 makes body 2
equation "d27 = 106 mm - 26 mm"
equation "d30 = 40 mm + ( 13 / 2 ) * 1 mm"
equation "d31 = 40 mm + ( 13 / 2 ) * 1 mm"
